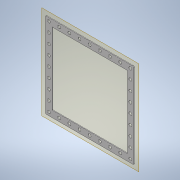
# Autodesk Inventor part: Деталь5
Saved by Autodesk Inventor 2021 (Build 250183000, 183)
## iProperties
Created: 2020-11-22
Part Number: Деталь5
Material: Алюминий 6061
Document SubType Name: Modeling
Designer: Тимоха
Mass: 93.8063 g
Surface Area: 404.628 cm^2
Volume: 34.7431 cm^3
Density: 2.7 g/cm^3
Appearance: Алюминий — плоский
Author: Тимоха
Autodesk Inventor part; units mm, degrees
ref_plane "YZ Plane" through (0, 0, 0) normal (1, 0, 0) x (0, 1, 0)
ref_plane "XZ Plane" through (0, 0, 0) normal (0, 1, 0) x (-1, 0, 0)
ref_plane "XY Plane" through (0, 0, 0) normal (0, 0, 1) x (1, 0, 0)
ref_plane "РабПлоскость1" through (0, 0, 0) normal (0, 0, 1) x (1, 0, 0)
sketch "Эскиз1" plane through (0, 0, 0) normal (0, 0, 1) x (1, 0, 0)
  circle A0 centre (124.164, -120) radius 4 projected
  circle A1 centre (93.064, -120) radius 4 projected
  circle A2 centre (61.964, -120) radius 4 projected
  circle A3 centre (30.864, -120) radius 4 projected
  circle A4 centre (-0.236, -120) radius 4 projected
  circle A5 centre (-31.336, -120) radius 4 projected
  circle A6 centre (-62.436, -120) radius 4 projected
  circle A7 centre (-93.536, -120) radius 4 projected
  circle A8 centre (-124.636, -120) radius 4 projected
  circle A9 centre (124.164, -90) radius 4 projected
  circle A10 centre (-124.636, -90) radius 4 projected
  circle A11 centre (124.164, -60) radius 4 projected
  circle A12 centre (-124.636, -60) radius 4 projected
  circle A13 centre (124.164, -30) radius 4 projected
  circle A14 centre (-124.636, -30) radius 4 projected
  circle A15 centre (124.164, 0) radius 4 projected
  circle A16 centre (-124.636, 0) radius 4 projected
  circle A17 centre (124.164, 30) radius 4 projected
  circle A18 centre (-124.636, 30) radius 4 projected
  circle A19 centre (124.164, 60) radius 4 projected
  circle A20 centre (-124.636, 60) radius 4 projected
  circle A21 centre (124.164, 90) radius 4 projected
  circle A22 centre (-124.636, 90) radius 4 projected
  circle A23 centre (124.164, 120) radius 4 projected
  circle A24 centre (93.064, 120) radius 4 projected
  circle A25 centre (61.964, 120) radius 4 projected
  circle A26 centre (30.864, 120) radius 4 projected
  circle A27 centre (-0.236, 120) radius 4 projected
  circle A28 centre (-31.336, 120) radius 4 projected
  circle A29 centre (-62.436, 120) radius 4 projected
  circle A30 centre (-93.536, 120) radius 4 projected
  circle A31 centre (-124.636, 120) radius 4 projected
  line L0 (115.364, 110) -> (115.364, -110) projected
  line L1 (115.364, -110) -> (-114.636, -110) projected
  line L2 (-114.636, -110) -> (-114.636, 110) projected
  line L3 (-114.636, 110) -> (115.364, 110) projected
  arc A32 (-132.636, 130) -> (-134.636, 128) centre (-132.636, 128) ccw projected
  line L4 (-134.636, 128) -> (-134.636, -128) projected
  arc A33 (-134.636, -128) -> (-132.636, -130) centre (-132.636, -128) ccw projected
  line L5 (-132.636, -130) -> (132.636, -130) projected
  arc A34 (132.636, -130) -> (134.636, -128) centre (132.636, -128) ccw projected
  line L6 (134.636, -128) -> (134.636, 128) projected
  arc A35 (134.636, 128) -> (132.636, 130) centre (132.636, 128) ccw projected
  line L7 (132.636, 130) -> (-132.636, 130) projected
  circle A36 centre (-124.636, 120) radius 4.5
  circle A37 centre (-93.536, 120) radius 4.5
  circle A38 centre (-62.436, 120) radius 4.5
  circle A39 centre (-31.336, 120) radius 4.5
  circle A40 centre (-0.236, 120) radius 4.5
  circle A41 centre (30.864, 120) radius 4.5
  circle A42 centre (61.964, 120) radius 4.5
  circle A43 centre (93.064, 120) radius 4.5
  circle A44 centre (124.164, 120) radius 4.5
  circle A45 centre (124.164, 90) radius 4.5
  circle A46 centre (124.164, 60) radius 4.5
  circle A47 centre (124.164, 30) radius 4.5
  circle A48 centre (124.164, 0) radius 4.5
  circle A49 centre (124.164, -30) radius 4.5
  circle A50 centre (124.164, -60) radius 4.5
  circle A51 centre (124.164, -90) radius 4.5
  circle A52 centre (124.164, -120) radius 4.5
  circle A53 centre (93.064, -120) radius 4.5
  circle A54 centre (61.964, -120) radius 4.5
  circle A55 centre (30.864, -120) radius 4.5
  circle A56 centre (-0.236, -120) radius 4.5
  circle A57 centre (-31.336, -120) radius 4.5
  circle A58 centre (-62.436, -120) radius 4.5
  circle A59 centre (-93.536, -120) radius 4.5
  circle A60 centre (-124.636, -120) radius 4.5
  circle A61 centre (-124.636, -90) radius 4.5
  circle A62 centre (-124.636, -60) radius 4.5
  circle A63 centre (-124.636, -30) radius 4.5
  circle A64 centre (-124.636, 0) radius 4.5
  circle A65 centre (-124.636, 30) radius 4.5
  circle A66 centre (-124.636, 60) radius 4.5
  circle A67 centre (-124.636, 90) radius 4.5
  point P0 (0, 0)
  dimension "d0" = 9
  dimension "d1" = 9
  dimension "d2" = 9
  dimension "d3" = 9
  dimension "d4" = 9
  dimension "d5" = 9
  dimension "d6" = 9
  dimension "d7" = 9
  dimension "d8" = 9
  dimension "d9" = 9
  dimension "d10" = 9
  dimension "d11" = 9
  dimension "d12" = 9
  dimension "d13" = 9
  dimension "d14" = 9
  dimension "d15" = 9
  dimension "d16" = 9
  dimension "d17" = 9
  dimension "d18" = 9
  dimension "d19" = 9
  dimension "d20" = 9
  dimension "d21" = 9
  dimension "d22" = 9
  dimension "d23" = 9
  dimension "d24" = 9
  dimension "d25" = 9
  dimension "d26" = 9
  dimension "d27" = 9
  dimension "d28" = 9
  dimension "d29" = 9
  dimension "d30" = 9
  dimension "d31" = 9
  constraints: 32 centre point, 32 coincident
  measures "d0" diameter of A36
  measures "d1" diameter of A37
  measures "d2" diameter of A38
  measures "d3" diameter of A39
  measures "d4" diameter of A40
  measures "d5" diameter of A41
  measures "d6" diameter of A42
  measures "d7" diameter of A43
  measures "d8" diameter of A44
  measures "d9" diameter of A45
  measures "d10" diameter of A46
  measures "d11" diameter of A47
  measures "d12" diameter of A48
  measures "d13" diameter of A49
  measures "d14" diameter of A50
  measures "d15" diameter of A51
  measures "d16" diameter of A52
  measures "d17" diameter of A53
  measures "d18" diameter of A54
  measures "d19" diameter of A55
  measures "d20" diameter of A56
  measures "d21" diameter of A57
  measures "d22" diameter of A58
  measures "d23" diameter of A59
  measures "d24" diameter of A60
  measures "d25" diameter of A61
  measures "d26" diameter of A62
  measures "d27" diameter of A63
  measures "d28" diameter of A64
  measures "d29" diameter of A65
  measures "d30" diameter of A66
  measures "d31" diameter of A67
extrude "Выдавливание1" add sketch "Эскиз1" along normal blind 2 contours L7 A35 L6 A34 L5 A33 L4 A32
